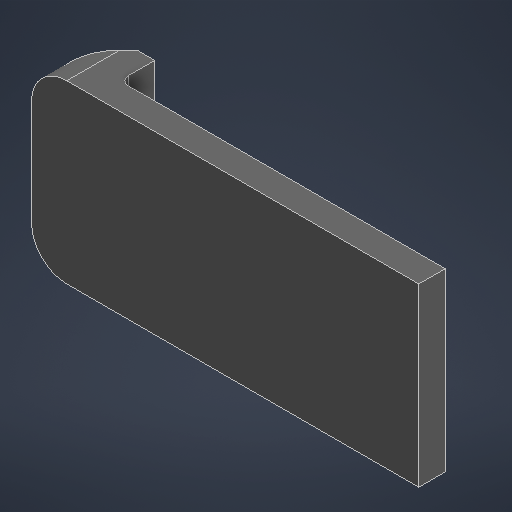
# Autodesk Inventor part: P_Wing_Mountingplate_pin
Saved by Autodesk Inventor 2026 (Build 300175000, 175)
## iProperties
Created: 2025-09-10
Part Number: P_Wing_Mountingplate_pin
Material: Generisch
Document SubType Name: Modeling
Designer: FAL
Density: 1 g/cm^3
Appearance: Vorgabe
Author: FAL
Autodesk Inventor part; units mm, degrees
ref_plane "YZ Plane" through (0, 0, 0) normal (1, 0, 0) x (0, 1, 0)
ref_plane "XZ Plane" through (0, 0, 0) normal (0, 1, 0) x (-1, 0, 0)
ref_plane "XY Plane" through (0, 0, 0) normal (0, 0, 1) x (1, 0, 0)
sketch "Skizze2" plane through (0, 0, 0) normal (0, 0, 1) x (1, 0, 0)
  line L0 (0, 0) -> (22, 0)
  line L1 (22, 0) -> (22, 1.5)
  line L2 (22, 1.5) -> (3.5, 1.5)
  line L3 (2.5, 3.5) -> (0, 1)
  line L4 (0, 1) -> (0, 0)
  line L5 (2.5, 3.5) -> (3.5, 3.5)
  line L6 (3.5, 3.5) -> (3.5, 1.5)
  dimension "d0" = 1.5
  dimension "d1" = 22
  dimension "d2" = 2
  dimension "d4" = 1
  dimension "d5" = 1
  dimension "d10" = 45
  constraints: 14 end point, 3 perpendicular, 2 horizontal, 1 parallel
  measures "d0" distance between parallel lines of L0 L2
  measures "d1" distance between parallel lines of L4 L1
  measures "d2" distance between parallel lines of L2 L5
  measures "d4" distance of L3.end L0.start
  measures "d5" distance of L3.start L5.end
  measures "d10" angle of L0 L3
extrude "Extrusion1" add sketch "Skizze2" along normal mid plane 10
fillet "Rundung1" radius 2 2 edges at (0, 0.5, 5) (0, 0.5, -5)
fillet "Rundung2" radius 0.5 1 edges at (3.5, 1.5, 0)
